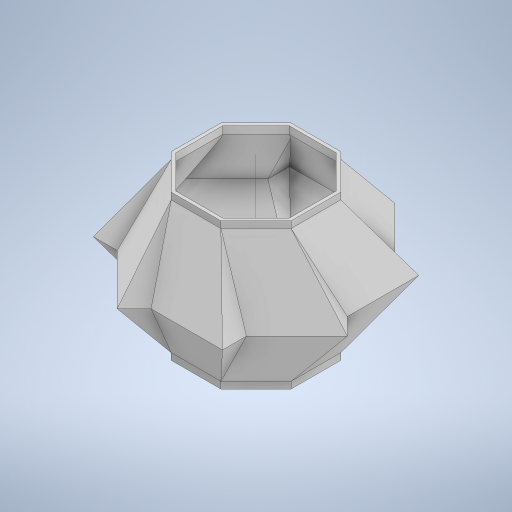
# Autodesk Inventor part: OV-PAM_tendon
Saved by Autodesk Inventor 2024 (Build 280153000, 153)
## iProperties
Created: 2023-07-13
Part Number: OV-PAM_tendon
Material: 일반
Document SubType Name: Modeling
Designer: jsw
Density: 1 g/cm^3
Appearance: 기본값
Author: jsw
Autodesk Inventor part; units mm, degrees
ref_plane "YZ Plane" through (0, 0, 0) normal (1, 0, 0) x (0, 1, 0)
ref_plane "XZ Plane" through (0, 0, 0) normal (0, 1, 0) x (-1, 0, 0)
ref_plane "XY Plane" through (0, 0, 0) normal (0, 0, 1) x (1, 0, 0)
sketch "스케치1" plane through (0, 0, 0) normal (0, 1, 0) x (-1, 0, 0)
  line L0 (10.864, -4.5) -> (4.5, -10.864)
  line L1 (4.5, -10.864) -> (-4.5, -10.864)
  line L2 (-4.5, -10.864) -> (-10.864, -4.5)
  line L3 (-10.864, -4.5) -> (-10.864, 4.5)
  line L4 (-10.864, 4.5) -> (-4.5, 10.864)
  line L5 (-4.5, 10.864) -> (4.5, 10.864)
  line L6 (4.5, 10.864) -> (10.864, 4.5)
  line L7 (10.864, 4.5) -> (10.864, -4.5)
  point P0 (0, 0)
  point P1 (0, 0)
  dimension "d0" = 9
  constraints: 16 end point, 1 coincident, 1 horizontal, 17 other
  measures "d0" distance of L6.end L0.start
extrude "돌출1" add sketch "스케치1" along normal blind 12
ref_plane "작업 평면5" through (-10.864, 0, -4.5) normal (-0.8660254, -0.5, 0) x (0, 0, 1)
sketch "스케치6" plane through (-10.864, 0, -4.5) normal (-1, 0, 0) x (0, 0, 1)
  line L0 (0, 0) -> (0, 12) projected
  line L1 (0, 0) -> (9, 0) projected
  line L2 (0, 0) -> (9, 0)
  line L3 (9, 0) -> (16.2103, 12)
  line L4 (9, 12) -> (15.364, 12) projected
  line L5 (0, 0) -> (1, 12)
  line L6 (0, 12) -> (9, 12) projected
  line L7 (16.2103, 12) -> (1, 12)
  line L8 (15.364, 12) -> (9, 12) projected
  point P0 (4.5, 0)
  dimension "d16" = 121
  dimension "d17" = 1
  constraints: 8 end point, 2 point on line, 1 collinear, 1 horizontal
  measures "d16" angle of L1 L3
  measures "d17" distance of L0.end L5.end
extrude "돌출5" add sketch "스케치6" along normal up to surface surface through (-10.864, 0, -4.5) normal (-0.8660254, -0.5, 0)
pattern_circular "원형 패턴3" count 8 over 360 about axis through (0, -10, 0) along (0, 1, 0) of "돌출5"
sketch "스케치7" plane through (0, 0, 0) normal (0, -1, 0) x (1, 0, 0)
  line L0 (-10.864, 4.5) -> (-4.5, 10.864) projected
  line L1 (-10.864, -4.5) -> (-10.864, 4.5) projected
  line L2 (-4.5, -10.864) -> (-10.864, -4.5) projected
  line L3 (4.5, -10.864) -> (-4.5, -10.864) projected
  line L4 (10.864, -4.5) -> (4.5, -10.864) projected
  line L5 (10.864, 4.5) -> (10.864, -4.5) projected
  line L6 (4.5, 10.864) -> (10.864, 4.5) projected
  line L7 (-4.5, 10.864) -> (4.5, 10.864) projected
  point P0 (0, 0)
extrude "돌출6" add sketch "스케치7" along normal blind 1.2
ref_plane "작업 평면6" through (0, 12, 0) normal (0, 1, 0) x (1, 0, 0)
mirror "미러2" about plane through (0, 12, 0) normal (0, 1, 0) of "돌출5", "원형 패턴3", "돌출6", "돌출1"
shell "쉘2" thickness 0.6 removed faces 2 at (-3.6213, 25.2, 1.5) at (-3.6213, -1.2, 1.5)
